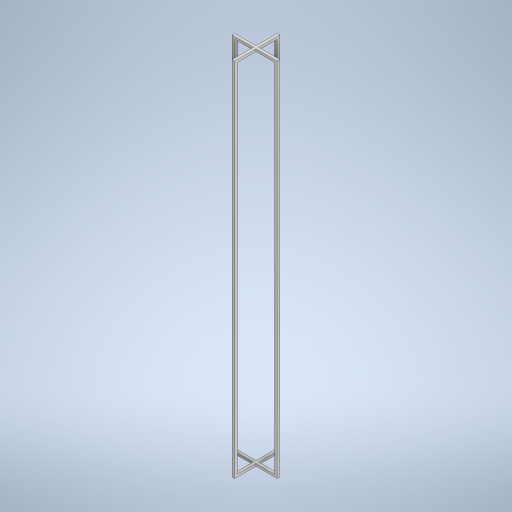
# Autodesk Inventor part: LigaXS
Saved by Autodesk Inventor 2024 (Build 280153000, 153)
## iProperties
Created: 2023-10-30
Part Number: LigaXS
Material: Genérico
Document SubType Name: Modeling
Designer: ismae
Density: 1 g/cm^3
Appearance: Valor por defecto
Author: ismae
Autodesk Inventor part; units mm, degrees
ref_plane "YZ Plane" through (0, 0, 0) normal (1, 0, 0) x (0, 1, 0)
ref_plane "XZ Plane" through (0, 0, 0) normal (0, 1, 0) x (-1, 0, 0)
ref_plane "XY Plane" through (0, 0, 0) normal (0, 0, 1) x (1, 0, 0)
sketch "Boceto1" plane through (0, 0, 0) normal (0, 1, 0) x (-1, 0, 0)
  circle A0 centre (0, 0) radius 13.1699
  line L0 (13.1485, 0.75) -> (-13.1485, 0.75)
  line L1 (-13.1485, 0.75) -> (-13.1485, -0.75)
  line L2 (-13.1485, -0.75) -> (13.1485, -0.75)
  line L3 (13.1485, -0.75) -> (13.1485, 0.75)
  line L4 (13.1485, 0.75) -> (-13.1485, -0.75) construction
  line L5 (-13.1485, 0.75) -> (13.1485, -0.75) construction
  line L6 (0.75, 13.1485) -> (-0.75, 13.1485)
  line L7 (-0.75, 13.1485) -> (-0.75, -13.1485)
  line L8 (0.75, -13.1485) -> (0.75, 13.1485)
  line L9 (-0.75, -13.1485) -> (0.75, -13.1485)
  line L10 (-13.1485, 0.75) -> (-13.1485, -0.75)
  line L11 (-13.1485, -0.75) -> (13.1485, -0.75)
  line L12 (13.1485, 0.75) -> (-13.1485, 0.75)
  line L13 (13.1485, -0.75) -> (13.1485, 0.75)
  line L14 (-0.75, -13.1485) -> (0.75, -13.1485)
  line L15 (0.75, -13.1485) -> (0.75, 13.1485)
  line L16 (-0.75, 13.1485) -> (-0.75, -13.1485)
  line L17 (0.75, 13.1485) -> (-0.75, 13.1485)
  point P0 (0.75, -0.75)
  point P1 (0.75, 0.75)
  point P2 (-0.75, 0.75)
  point P3 (-0.75, -0.75)
  dimension "d0" = 26.3398
  dimension "d1" = 1.5
  dimension "d4" = 360
  constraints: 36 end point, 2 midpoint, 2 parallel, 1 coincident, 1 horizontal, 1 perpendicular, 36 other
  measures "d1" distance of L1.end L0.end
extrude "Extrusión1" add sketch "Boceto1" along normal blind 210.82 contours L3 L2 L8 L0 | L8 L0 L7 L6 | L8 L2 L7 L0 | L9 L7 L2 L8 | L7 L2 L1 L0
sketch "Boceto2" plane through (0, 210.82, 0) normal (0, 1, 0) x (1, 0, 0)
  circle A0 centre (0, 0) radius 11.5572
  constraints: 1 centre point, 1 coincident
ref_plane "Plano de trabajo1" through (0, 105.41, 0) normal (0, 1, 0) x (1, 0, 0)
sketch "Boceto3" plane through (0, 105.41, 0) normal (0, 1, 0) x (1, 0, 0)
  circle A0 centre (0, 0) radius 11.5984
  constraints: 1 centre point, 1 coincident
extrude "Extrusión2" cut sketch "Boceto3" along normal mid plane 207.9625
